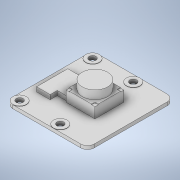
# Autodesk Inventor part: RasCamera
Saved by Autodesk Inventor 2022 (Build 260153000, 153)
## iProperties
Created: 2022-05-30
Part Number: RasCamera
Material: 일반
Document SubType Name: Modeling
Designer: user
Density: 1 g/cm^3
Appearance: 기본값
Author: user
Autodesk Inventor part; units mm, degrees
ref_plane "YZ Plane" through (0, 0, 0) normal (1, 0, 0) x (0, 1, 0)
ref_plane "XZ Plane" through (0, 0, 0) normal (0, 1, 0) x (-1, 0, 0)
ref_plane "XY Plane" through (0, 0, 0) normal (0, 0, 1) x (1, 0, 0)
sketch "스케치1" plane through (0, 0, 0) normal (0, 0, 1) x (1, 0, 0)
  line L0 (-12.75, -12) -> (12.75, -12)
  line L1 (12.75, -12) -> (12.75, 12)
  line L2 (12.75, 12) -> (-12.75, 12)
  line L3 (-12.75, 12) -> (-12.75, -12)
  line L4 (-12.75, -12) -> (12.75, 12) construction
  line L5 (12.75, -12) -> (-12.75, 12) construction
  line L6 (-4.25, 2.8) -> (4.25, 2.8)
  line L7 (4.25, 2.8) -> (4.25, -5.7)
  line L8 (4.25, -5.7) -> (-4.25, -5.7)
  line L9 (-4.25, -5.7) -> (-4.25, 2.8)
  line L10 (-4.25, 2.8) -> (4.25, -5.7) construction
  line L11 (4.25, 2.8) -> (-4.25, -5.7) construction
  line L12 (-5.95, 9.8) -> (3.25, 9.8)
  line L13 (3.25, 9.8) -> (3.25, 5.8)
  line L14 (3.25, 5.8) -> (-5.95, 5.8)
  line L15 (-5.95, 5.8) -> (-5.95, 9.8)
  line L16 (3.25, 9.8) -> (-3.85, 9.8)
  line L17 (-3.85, 9.8) -> (-3.85, 2.8)
  line L18 (-3.85, 2.8) -> (3.25, 2.8)
  line L19 (3.25, 2.8) -> (3.25, 9.8)
  circle A0 centre (-10.75, 10) radius 1
  point P0 (0, 0)
  point P1 (0, -1.45)
  point P2 (3.25, 2.8)
  point P3 (-3.85, 5.8)
  point P4 (0, -1.45)
  point P5 (0, 0)
  dimension "d0" = 25.5
  dimension "d1" = 24
  dimension "d2" = 8.5
  dimension "d3" = 8.5
  dimension "d4" = 17.7
  dimension "d5" = 1
  dimension "d6" = 7.1
  dimension "d7" = 4
  dimension "d8" = 7
  dimension "d9" = 9.2
  dimension "d10" = 2
  dimension "d11" = 2
  dimension "d12" = 2
  constraints: 40 end point, 8 parallel, 6 midpoint, 4 horizontal, 4 perpendicular, 1 centre point, 1 point on line, 1 vertical alignment
  measures "d0" distance of L2.end L1.end
  measures "d1" distance of L1.end L0.end
  measures "d2" distance of L7.end L8.end
  measures "d3" distance of L6.end L7.end
  measures "d4" distance between parallel lines of L2 L8
  measures "d5" distance between parallel lines of L7 L19
  measures "d6" distance of L12.end L16.end
  measures "d7" distance of L14.end L12.start
  measures "d8" distance between parallel lines of L6 L16
  measures "d9" distance of L12.start L12.end
  measures "d10" diameter of A0
  measures "d11" distance from line of L2 A0.centre
  measures "d12" distance from line of L3 A0.centre
extrude "돌출1" add sketch "스케치1" against normal blind 1 contours L3 L2 L1 L0 | L6 L7 L8 L9 | L17 L14 L19 L6 | L17 L12 L13 L14 | L14 L15 L12 L17 | A0
extrude "돌출2" cut sketch "스케치1" against normal blind 1 contours A0
extrude "돌출3" add sketch "스케치1" along normal blind 1.3 contours L17 L14 L19 L6 | L17 L12 L13 L14 | L14 L15 L12 L17
extrude "돌출4" add sketch "스케치1" along normal blind 3.3 contours L6 L7 L8 L9
fillet "모깎기1" radius 2 4 edges at (-12.75, 12, -0.5) (-12.75, -12, -0.5) (12.75, -12, -0.5) (12.75, 12, -0.5)
mirror "미러3" about plane through (0, 0, 0) normal (1, 0, 0) of "돌출2"
pattern_linear "직사각형 패턴1" count 2 spacing 12 along (0, -1, 0) of "돌출2", "미러3"
sketch "스케치2" plane through (0, 0, 0) normal (0, 0, 1) x (1, 0, 0)
  point P0 (0, 0)
sketch "스케치3" plane through (0, 0, 3.3) normal (0, 0, 1) x (1, 0, 0)
  line L0 (3.25, 2.8) -> (4.25, 2.8) projected
  line L1 (-4.25, -5.7) -> (4.25, -5.7) projected
  line L2 (4.25, 2.8) -> (-4.25, -5.7) construction
  circle A0 centre (0, -1.45) radius 3.75
  line L3 (4.25, 2.8) -> (-4.25, 2.8) projected
  line L4 (-4.25, 2.8) -> (-3.25, 2.8)
  line L5 (-3.25, 2.8) -> (-3.25, 2.1)
  line L6 (-3.55, 1.8) -> (-4.25, 1.8)
  line L7 (-4.25, 1.8) -> (-4.25, 2.8)
  line L8 (4.25, 2.8) -> (3.25, 2.8)
  line L9 (3.25, 2.8) -> (3.25, 2.1)
  line L10 (3.55, 1.8) -> (4.25, 1.8)
  line L11 (4.25, 1.8) -> (4.25, 2.8)
  line L12 (0, -1.45) -> (2.1267, -1.45) construction
  line L13 (3.25, -5.7) -> (4.25, -5.7)
  line L14 (4.25, -5.7) -> (-4.25, -5.7)
  line L15 (-3.25, -5.7) -> (-3.25, -5)
  line L16 (-3.55, -4.7) -> (-4.25, -4.7)
  line L17 (-4.25, -4.7) -> (-4.25, -5.7)
  line L18 (3.25, -5.7) -> (3.25, -5)
  line L19 (3.55, -4.7) -> (4.25, -4.7)
  line L20 (4.25, -4.7) -> (4.25, -5.7)
  arc A1 (-3.55, 1.8) -> (-3.25, 2.1) centre (-3.55, 2.1) ccw
  arc A2 (3.25, 2.1) -> (3.55, 1.8) centre (3.55, 2.1) ccw
  arc A3 (3.55, -4.7) -> (3.25, -5) centre (3.55, -5) ccw
  arc A4 (-3.25, -5) -> (-3.55, -4.7) centre (-3.55, -5) ccw
  point P0 (0, 0)
  point P1 (-3.25, 1.8)
  point P2 (3.25, 1.8)
  point P3 (-3.25, -4.7)
  point P4 (3.25, -4.7)
  dimension "d25" = 7.5
  dimension "d26" = 1
  dimension "d27" = 1
  dimension "d28" = 1
  dimension "d31" = 0.3
  constraints: 36 end point, 9 point on line, 8 point on circle, 8 tangent, 7 symmetric about line, 5 centre point, 4 parallel, 3 equal radius, 2 horizontal, 2 perpendicular, 1 midpoint
  measures "d25" diameter of A0
  measures "d26" distance of point (-3.25, 1.8) L6.end
  measures "d27" distance of L10.end point (3.25, 1.8)
  measures "d28" distance of L4.end point (-3.25, 1.8)
  measures "d31" radius of A1
extrude "돌출5" add sketch "스케치3" along normal blind 2.5 contours A0
extrude "돌출6" cut sketch "스케치3" against normal blind 0.2 contours L0 L11 L10 A2 L9 | L17 L16 A4 L15 L1 | L18 A3 L19 L20 L1 | L5 A1 L6 L7 L3
sketch "스케치4" plane through (0, 0, 0) normal (0, 0, 1) x (1, 0, 0)
  circle A0 centre (-10.75, 10) radius 1 projected
  arc A1 (-10.75, 12) -> (-12.75, 10) centre (-10.75, 10) ccw projected
  circle A2 centre (-10.75, 10) radius 2
  circle A3 centre (10.75, 10) radius 1 projected
  line L0 (10.75, 12) -> (-10.75, 12) projected
  circle A4 centre (10.75, 10) radius 2
  circle A5 centre (10.75, -2) radius 1 projected
  circle A6 centre (10.75, -2) radius 2
  circle A7 centre (-10.75, -2) radius 2
  line L1 (-12.75, 10) -> (-12.75, -10) projected
  circle A8 centre (-10.75, -2) radius 1 projected
  point P0 (0, 0)
  point P1 (-12.75, 10)
  constraints: 3 coincident, 2 centre point, 1 tangent, 1 vertical alignment, 5 other
extrude "돌출7" add sketch "스케치4" along normal blind 0.1
